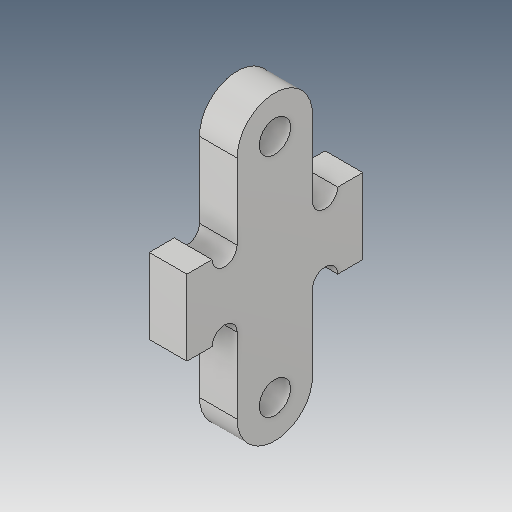
# Autodesk Inventor part: tip
Saved by Autodesk Inventor 2019.4 (Build 234330000, 330)
## iProperties
Created: 2019-06-11
Part Number: tip
Material: アルミニウム 2014-T4
Document SubType Name: Modeling
Designer: AzLIer
Density: 2.8 g/cm^3
Appearance: サテン
Mass: 1.41266 g
Surface Area: 6.09719 cm^2
Volume: 0.504521 cm^3
Author: AzLIer
Autodesk Inventor part; units mm, degrees
note: some values were not read from the file. Chosen so that the rebuilt part matches the saved one: sketch regions of "押し出し1".
ref_plane "YZ Plane" through (0, 0, 0) normal (1, 0, 0) x (0, 1, 0)
ref_plane "XZ Plane" through (0, 0, 0) normal (0, 1, 0) x (-1, 0, 0)
ref_plane "XY Plane" through (0, 0, 0) normal (0, 0, 1) x (1, 0, 0)
sketch "スケッチ1" plane through (0, 0, 0) normal (1, 0, 0) x (0, 1, 0)
  line L0 (9, 0) -> (-9, 0) construction
  line L1 (9, 3) -> (-9, 3)
  line L2 (-9, -3) -> (9, -3)
  arc A0 (9, -3) -> (9, 3) centre (9, 0) ccw
  arc A1 (-9, 3) -> (-9, -3) centre (-9, 0) ccw
  line L3 (3, 7) -> (-3, 7)
  line L4 (-3, -7) -> (3, -7)
  line L5 (3, 7) -> (-3, -7) construction
  line L6 (-3, 7) -> (3, -7) construction
  arc A2 (3, 5) -> (3, 3) centre (3, 4) ccw
  arc A3 (-3, 3) -> (-3, 5) centre (-3, 4) ccw
  arc A4 (-3, -5) -> (-3, -3) centre (-3, -4) ccw
  arc A5 (3, -3) -> (3, -5) centre (3, -4) ccw
  line L7 (-3, 7) -> (-3, 5)
  line L8 (3, 5) -> (3, 7)
  line L9 (3, -7) -> (3, -5)
  line L10 (3, -3) -> (3, 3)
  line L11 (-3, 3) -> (-3, -3)
  line L12 (-3, -5) -> (-3, -7)
  circle A6 centre (-9, 0) radius 1.25
  circle A7 centre (9, 0) radius 1.25
  point P0 (0, 0)
  dimension "d0" = 6
  dimension "d1" = 6
  dimension "d2" = 1
  dimension "d3" = 14
  dimension "d4" = 18
  dimension "d7" = 0
  dimension "d8" = 6
  dimension "d9" = 4
  dimension "d10" = 6
  dimension "d11" = 2.5
  dimension "d12" = 2.5
  constraints: 28 end point, 12 point on circle, 11 parallel, 8 centre point, 8 tangent, 3 equal radius, 3 midpoint, 3 perpendicular, 2 coincident, 2 collinear, 2 horizontal, 2 point on line
  measures "d0" diameter of A1
  measures "d1" distance of L4.start L4.end
  measures "d2" radius of A2
  measures "d3" distance between parallel lines of L4 L3
  measures "d4" distance of L0.start L0.end
  measures "d7" distance between parallel lines of L8 L10
  measures "d8" distance between parallel lines of L8 L11
  measures "d9" distance from line of L10.start L4
  measures "d10" distance from line of A4.centre L8
  measures "d11" diameter of A6
  measures "d12" diameter of A7
extrude "押し出し1" add sketch "スケッチ1" along normal blind 3
